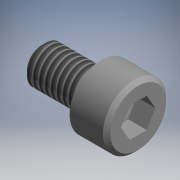
# Autodesk Inventor part: CB5-8
Saved by Autodesk Inventor 2017.3 (Build 213256000, 256)
## iProperties
Part Number: CB5-8
Material: Generic
Catalog Web Link: www.cadenas.de
Description: CB-Hexagon Socket Head Cap Screws
Vendor: MISUMI
Document SubType Name: Modeling
Designer: partserver
Manufacturer: MISUMI
Mass: 0.398946 g
Surface Area: 3.94783 cm^2
Volume: 0.398946 cm^3
Density: 1 g/cm^3
Appearance: PSOLRGB-175-175-175
Category: PARTsolutions
Company: MISUMI
Title: CB5-8
Author: Cadenas PARTsolutions
Comments: Hexagon Socket Head Cap Screws
PSOL_IDENT_0: {$CADENAS_DATA\23d-libs\misumi\metric\27_screws_nuts\cb_fa.prj},148 {VTYP=3D},{NB=CB5-8},{LINA=CB5-8
PSOL_IDENT_1: },{NN=CB},{DATE=30.06.2021 13:09:25},{GEOMDATE=17.02.2014 00:00:00},{VERSION=},{LINEID=40},{WBVAR=L}
PSOL_IDENT_2: ,{WBNUMERIC=L}  {NB=CB5-8},{LINA=CB5-8},{KT=DUMMY},{PN=CB5-8},{MAT=4137 Steel},{HARD=38~43HRC},{ST=B
PSOL_IDENT_3: lack Oxide},{M=5},{L=8},{LL=Full Thread},{L1=22},{TYPE=CB},{M1=5.000},{L0=5,6,8,10,12,14,15,16,18,20
PSOL_IDENT_4: ,22,25,30,35,40,45,50,55,60,65,70,75,80},{NDM=5},{KDM=4.017064},{MP=5x0.8},{P=0.8},{A=8.5},{E=5.0},{
PSOL_IDENT_5: B=4.0},{V=0.5}
NB: CB5-8
NN: CB
NT: Hexagon Socket Head Cap Screws
NBSYN: $PN.
LINA: CB5-8
CATALOG: Misumi
PN: CB5-8
MAT: 4137 Steel
HARD: 38~43HRC
ST: Black Oxide
M: 5
L: 8
LL: Full Thread
MP: 5x0.8
A: 8.5
E: 5
B: 4
SUPPLIER: MISUMI
ARTICLENO: CB5-8
BOMINFO: CB5-8
CREATOR: CADENAS GmbH
Autodesk Inventor part; units mm, degrees
sketch "Sketch_1" plane through (0, 0, 0) normal (0, 0, 1) x (1, 0, 0)
  line L0 (8, 0) -> (-5, 0)
  line L1 (-5, 0) -> (-5, 3.75)
  line L2 (-5, 3.75) -> (-4.5, 4.25)
  line L3 (-4.5, 4.25) -> (0, 4.25)
  line L4 (0, 4.25) -> (0, 2.5)
  line L5 (0, 2.5) -> (7.5095, 2.5)
  line L6 (7.5095, 2.5) -> (8, 2.0095)
  line L7 (8, 2.0095) -> (8, 0)
  line L8 (8, 0) -> (-5, 0)
  constraints: 18 end point
revolve "Revolution1" add sketch "Sketch_1" angle 360 about axis through (8, 0, 0) along (1, 0, 0)
thread "Thread1" size "M5x0.8" class "6g" standard "ISO Metric profile" length 6.5095
sketch "Sketch2" plane through (-5, 0, 0) normal (-1, 0, 0) x (0, 0, 1)
  point P0 (0, 0)
hole "Hole1" at (-5, 0, 0) direction (1, 0, 0) diameter 4 depth 2.5 tip angle 150
sketch "Sketch_3" plane through (-5, 0, 0) normal (1, 0, 0) x (0, 0, -1)
  line L0 (-2, -1.1547) -> (0, -2.3094)
  line L1 (0, -2.3094) -> (2, -1.1547)
  line L2 (2, -1.1547) -> (2, 1.1547)
  line L3 (2, 1.1547) -> (0, 2.3094)
  line L4 (0, 2.3094) -> (-2, 1.1547)
  line L5 (-2, 1.1547) -> (-2, -1.1547)
  constraints: 12 end point
extrude "Extrusion1" cut sketch "Sketch_3" along normal blind 2.5
ref_plane "bolt_to_nut_XY" through (8, 0, 0) normal (1, 0, 0) x (0, 0, -1)
ref_plane "bolt_to_nut_YZ" through (8, 0, 0) normal (0, 0, -1) x (0, 1, 0)
ref_plane "bolt_to_nut_ZX" through (8, 0, 0) normal (0, 1, 0) x (1, 0, 0)
ref_plane "screw1_XY" through (0, 0, 0) normal (1, 0, 0) x (0, 0, -1)
ref_plane "screw1_YZ" through (0, 0, 0) normal (0, 0, -1) x (0, 1, 0)
ref_plane "screw1_ZX" through (0, 0, 0) normal (0, 1, 0) x (1, 0, 0)
body "Solid1"
